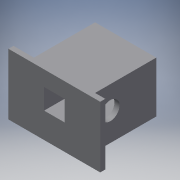
# Autodesk Inventor part: krytymotor
Saved by Autodesk Inventor 2016 (Build 200138000, 138)
## iProperties
Created: 2015-06-19
Part Number: krytymotor
Material: Generic
Document SubType Name: Modeling
Designer: Jufo
Density: 1 g/cm^3
Appearance: Default
Author: Jufo
Autodesk Inventor part; units mm, degrees
ref_plane "YZ Plane" through (0, 0, 0) normal (1, 0, 0) x (0, 1, 0)
ref_plane "XZ Plane" through (0, 0, 0) normal (0, 1, 0) x (-1, 0, 0)
ref_plane "XY Plane" through (0, 0, 0) normal (0, 0, 1) x (1, 0, 0)
sketch "Sketch1" plane through (0, 0, 0) normal (0, 1, 0) x (-1, 0, 0)
  line L0 (-6.1909, 7.7955) -> (5.8091, 7.7955)
  line L1 (5.8091, 7.7955) -> (5.8091, -2.2045)
  line L2 (5.8091, -2.2045) -> (-6.1909, -2.2045)
  line L3 (-6.1909, -2.2045) -> (-6.1909, 7.7955)
  point P0 (0, 0)
  dimension "d0" = 12
  dimension "d1" = 10
  constraints: 8 end point, 2 parallel, 1 horizontal, 1 perpendicular
  measures "d0" distance of L0.start L0.end
  measures "d1" distance of L0.end L1.end
extrude "Extrusion1" add sketch "Sketch1" along normal blind 13
sketch "Sketch2" plane through (6.1909, 0, 7.7955) normal (1, 0, 0) x (0, 0, -1)
  line L0 (10, 0) -> (0, 0) projected
  line L1 (10, 0) -> (10, 13) projected
  line L2 (0, 0) -> (0, 13) projected
  circle A0 centre (4.5, 4) radius 1.8
  point P0 (7.7955, 0)
  dimension "d4" = 3.6
  dimension "d5" = 4
  dimension "d7" = 5.5
  dimension "d8" = 4.5
  constraints: 1 centre point
  measures "d4" diameter of A0
  measures "d5" distance from line of L0 A0.centre
  measures "d7" distance from line of L1 A0.centre
  measures "d8" distance from line of L2 A0.centre
extrude "Extrusion2" cut sketch "Sketch2" against normal blind 13
sketch "Sketch3" plane through (0, 0, 0) normal (0, -1, 0) x (1, 0, 0)
  line L0 (6.1909, 7.7955) -> (-5.8091, 7.7955) projected
  line L1 (-5.8091, 7.7955) -> (-5.8091, -2.2045) projected
  line L2 (-5.8091, -2.2045) -> (6.1909, -2.2045) projected
  line L3 (6.1909, -2.2045) -> (6.1909, 7.7955) projected
  line L4 (-4.8091, 6.7955) -> (-4.8091, -1.2045)
  line L5 (-4.8091, -1.2045) -> (5.1909, -1.2045)
  line L6 (5.1909, -1.2045) -> (5.1909, 6.7955)
  line L7 (5.1909, 6.7955) -> (-4.8091, 6.7955)
  point P0 (0, 0)
  dimension "d11" = 1
  dimension "d12" = 1
  dimension "d14" = 1
  dimension "d15" = 1
  constraints: 8 end point, 3 parallel, 1 perpendicular
  measures "d11" distance between parallel lines of L1 L4
  measures "d12" distance between parallel lines of L0 L7
  measures "d14" distance between parallel lines of L3 L6
  measures "d15" distance between parallel lines of L2 L5
extrude "Extrusion3" cut sketch "Sketch3" against normal blind 13 contours L7 L6 L5 L4
sketch "Sketch4" plane through (0, 0, 0) normal (0, -1, 0) x (1, 0, 0)
  line L0 (6.1909, 7.7955) -> (-5.8091, 7.7955) projected
  line L1 (-5.8091, 7.7955) -> (-5.8091, -2.2045) projected
  line L2 (-5.8091, -2.2045) -> (6.1909, -2.2045) projected
  line L3 (6.1909, -2.2045) -> (6.1909, 7.7955) projected
  line L4 (-8.8091, 8.7955) -> (-8.8091, -3.2045)
  line L5 (-8.8091, -3.2045) -> (9.1909, -3.2045)
  line L6 (9.1909, -3.2045) -> (9.1909, 8.7955)
  line L7 (9.1909, 8.7955) -> (-8.8091, 8.7955)
  point P0 (0, 0)
  dimension "d18" = 3
  dimension "d19" = 3
  dimension "d20" = 1
  dimension "d21" = 1
  dimension "d34" = 18
  dimension "d35" = 12
  dimension "d36" = 12
  constraints: 8 end point, 3 parallel, 1 perpendicular
  measures "d18" distance between parallel lines of L4 L1
  measures "d19" distance between parallel lines of L6 L3
  measures "d20" distance between parallel lines of L7 L0
  measures "d21" distance between parallel lines of L5 L2
  measures "d34" distance between parallel lines of L6 L4
  measures "d35" distance between parallel lines of L5 L7
  measures "d36" distance between parallel lines of L3 L1
extrude "Extrusion4" add sketch "Sketch4" along normal blind 1 contours L3 L2 L1 L0 | L7 L6 L5 L4
sketch "Sketch5" plane through (0, -1, 0) normal (0, -1, 0) x (1, 0, 0)
  line L0 (9.1909, -3.2045) -> (9.1909, 8.7955) projected
  line L1 (9.1909, 8.7955) -> (-8.8091, 8.7955) projected
  line L2 (0.1909, 5.7955) -> (2.1909, 5.7955)
  line L3 (2.1909, 5.7955) -> (2.1909, 1.7955)
  line L4 (2.1909, 1.7955) -> (-1.8091, 1.7955)
  line L5 (-1.8091, 1.7955) -> (-1.8091, 5.7955)
  line L6 (-1.8091, 5.7955) -> (2.1909, 5.7955)
  point P0 (0, 0)
  dimension "d27" = 2
  dimension "d28" = 4
  dimension "d29" = 4
  dimension "d30" = 3
  dimension "d31" = 9
  constraints: 10 end point, 2 parallel, 1 collinear, 1 perpendicular
  measures "d27" distance of L2.start L2.end
  measures "d28" distance of L2.end L3.end
  measures "d29" distance of L3.end L4.end
  measures "d30" distance between parallel lines of L1 L6
  measures "d31" distance from line of L0 L2.start
extrude "Extrusion5" cut sketch "Sketch5" against normal blind 1
body "Solid1"
